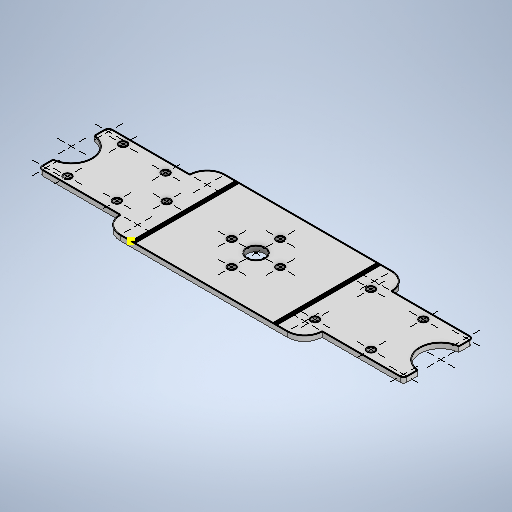
# Autodesk Inventor part: axis_19_top_frame
Saved by Autodesk Inventor 2025.2 (Build 292293000, 293)
## iProperties
Created: 2025-08-10
Part Number: axis_19_top_frame
Material: Generic
Document SubType Name: Modeling
Designer: LG
Density: 1 g/cm^3
Appearance: Default
Author: LG
Autodesk Inventor part; units mm, degrees
ref_plane "YZ Plane" through (0, 0, 0) normal (1, 0, 0) x (0, 1, 0)
ref_plane "XZ Plane" through (0, 0, 0) normal (0, 1, 0) x (-1, 0, 0)
ref_plane "XY Plane" through (0, 0, 0) normal (0, 0, 1) x (1, 0, 0)
sketch "Sketch1" plane through (0, 0, 0) normal (0, 1, 0) x (-1, 0, 0)
  line L0 (-0.4496, -30) -> (-0.4496, 0)
  line L1 (-41.2289, 0) -> (-41.2289, -30)
  circle A0 centre (-20.8393, -15) radius 2.6
  circle A1 centre (-61.4686, -7.475) radius 1.05
  circle A2 centre (-61.4686, -22.525) radius 1.05
  circle A3 centre (-45.8686, -6.93) radius 1.05
  circle A4 centre (-46.3686, -22.525) radius 1.05
  circle A5 centre (4.87, -15) radius 1.05
  circle A6 centre (12.17, -8) radius 1.05
  circle A7 centre (25.39, -7) radius 1.05
  circle A8 centre (12.17, -22) radius 1.05
  circle A9 centre (25.39, -23) radius 1.05
  circle A10 centre (-27.8393, -15) radius 1.05
  circle A11 centre (-20.8393, -8) radius 1.05
  circle A12 centre (-20.8393, -22) radius 1.05
  circle A13 centre (-13.8393, -15) radius 1.05
  arc A14 (-72.2686, -5) -> (-73.2686, -6) centre (-72.2686, -6) ccw
  line L2 (-73.2686, -9.041) -> (-73.2686, -6)
  arc A15 (31.59, -6) -> (30.59, -5) centre (30.59, -6) ccw
  line L3 (31.59, -6) -> (31.59, -9.041)
  arc A16 (30.59, -25) -> (31.59, -24) centre (30.59, -24) ccw
  line L4 (8.19, -25) -> (30.59, -25)
  arc A17 (-73.2686, -24) -> (-72.2686, -25) centre (-72.2686, -24) ccw
  line L5 (-73.2686, -24) -> (-73.2686, -20.959)
  arc A18 (-73.2686, -20.959) -> (-73.2686, -9.041) centre (-73.9686, -15) ccw
  line L6 (-72.2686, -25) -> (-49.8686, -25)
  arc A19 (-49.8686, -25) -> (-44.8686, -30) centre (-44.8686, -25) ccw
  line L7 (3.19, -30) -> (-44.8686, -30)
  arc A20 (3.19, -30) -> (8.19, -25) centre (3.19, -25) ccw
  line L8 (31.59, -20.959) -> (31.59, -24)
  arc A21 (31.59, -9.041) -> (31.59, -20.959) centre (32.29, -15) ccw
  line L9 (30.59, -5) -> (8.19, -5)
  arc A22 (8.19, -5) -> (3.19, 0) centre (3.19, -5) ccw
  line L10 (-44.8686, 0) -> (3.19, 0)
  arc A23 (-44.8686, 0) -> (-49.8686, -5) centre (-44.8686, -5) ccw
  line L11 (-49.8686, -5) -> (-72.2686, -5)
  line L12 (-41.6786, -30) -> (-41.6786, 0)
  line L13 (-40.7793, 0) -> (-40.7793, -30)
  line L14 (-0.8993, -30) -> (-0.8993, 0)
  line L15 (0, 0) -> (0, -30)
  constraints: 32 end point, 24 centre point, 20 point on circle, 20 tangent, 19 equal radius, 12 point on line, 10 vertical, 7 parallel, 6 horizontal, 4 perpendicular, 81 other
extrude "Extrusion1" add sketch "Sketch1" against normal blind 1.5
body "Solid1"
